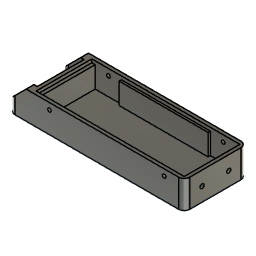
Upper Case v1 (Autodesk Fusion 360 design; units mm, degrees)
Autodesk Fusion 360 part; units mm, degrees
sketch "Sketch1" plane through (0, 0, 0) normal (0, 0, 1) x (1, 0, 0)
  line L0 (0, 0) -> (133, 0)
  line L1 (133, 0) -> (133, -56)
  line L2 (133, -56) -> (0, -56)
  line L3 (0, -56) -> (0, 0)
  dimension "d1" = 133
  dimension "d2" = 56
  constraint horizontal L0
  constraint vertical L1
  constraint horizontal L2
  constraint vertical L3
  constraint coincident L0.start L3.end
  measures "d1" distance of L0.start L0.end
  measures "d2" distance of L0.start L2.end
extrude "Extrude1" add sketch "Sketch1" along normal blind 3
sketch "Sketch2" plane through (0, 0, 3) normal (0, 0, 1) x (-1, 0, 0)
  line L0 (0, 56) -> (-133, 56)
  line L1 (-133, 56) -> (-133, 0)
  line L2 (-133, 0) -> (0, 0)
  line L3 (0, 0) -> (0, 56)
  line L4 (-3, 3) -> (-136, 3)
  line L5 (-136, 3) -> (-136, 53)
  line L6 (-136, 53) -> (-3, 53)
  line L7 (-3, 53) -> (-3, 3)
  dimension "d5" = 133
  dimension "d6" = 50
  dimension "d7" = 3
  dimension "d8" = 3
  constraint horizontal L4
  constraint vertical L5
  constraint horizontal L6
  constraint vertical L7
  measures "d5" distance of L4.start L4.end
  measures "d6" distance of L4.start L6.end
  measures "d7" distance of L2 L4
  measures "d8" distance of L3 L7
move_face "OffsetFaces1" offset 6 1 faces at (133, -18.6667, 1)
extrude "Extrude2" add sketch "Sketch2" along normal blind 22 contours L0 L1 L2 L3 L4 L6 L7
sketch "Sketch3" plane through (0, 0, 3) normal (0, 0, 1) x (-1, 0, 0)
  line L0 (-133, 0) -> (-133, 3)
  line L1 (-133, 3) -> (-3, 3)
  line L2 (-3, 3) -> (-3, 53)
  line L3 (-3, 53) -> (-133, 53)
  line L4 (-133, 53) -> (-133, 56)
  line L5 (-133, 56) -> (-139, 56)
  line L6 (-139, 56) -> (-139, 0)
  line L7 (-139, 0) -> (-133, 0)
  line L8 (-139, 0) -> (-136, 0)
  line L9 (-136, 0) -> (-136, 56)
  line L10 (-136, 56) -> (-139, 56)
  line L11 (-139, 56) -> (-139, 0)
  constraint horizontal L8
  constraint vertical L9
  constraint horizontal L10
  constraint vertical L11
  constraint midpoint L5 L9.end
  constraint coincident L6.end L7.start
extrude "Extrude3" add sketch "Sketch3" along normal blind 22 contours L5 L6 L7 L8 L9 L10 L11
move_face "OffsetFaces2" offset 5 1 faces at (133, -55, 10.3333)
move_face "OffsetFaces3" offset 5 1 faces at (133, -1, 17.6667)
sketch "Sketch4" plane through (0, 0, 0) normal (0, 1, 0) x (-1, 0, 0)
  line L0 (0, 25) -> (-139, 25)
  line L1 (-139, 25) -> (-139, 0)
  line L2 (-139, 0) -> (0, 0)
  line L3 (0, 0) -> (0, 25)
  line L4 (-136, 31.9366) -> (-136, -10) construction
  line L5 (-3, 30) -> (-3, -10) construction
  line L6 (-121, 35.1496) -> (-121, -13.3371) construction
  line L7 (-18, 34.1272) -> (-18, -18.3027) construction
  line L8 (-146.6322, 22) -> (13.2863, 22) construction
  line L9 (-145.902, 19.25) -> (3.6473, 19.25) construction
  point P0 (-121, 19.25)
  point P1 (-18, 19.25)
  dimension "d16" = 3
  dimension "d17" = 3
  dimension "d18" = 15
  dimension "d19" = 15
  dimension "d20" = 3
  dimension "d21" = 2.75
  constraint perpendicular L2 L4
  constraint perpendicular L2 L5
  constraint perpendicular L2 L6
  constraint perpendicular L0 L7
  constraint perpendicular L6 L8
  constraint perpendicular L3 L9
  constraint coincident L6 P0
  constraint coincident L9 P0
  constraint coincident L7 P1
  constraint coincident L9 P1
  measures "d16" distance of L1 L4
  measures "d17" distance of L3 L5
  measures "d18" distance of L4 L6
  measures "d19" distance of L5 L7
  measures "d20" distance of L0 L8
  measures "d21" distance of L8 L9
hole "Hole1" at (121, 0, 19.25) at (18, 0, 19.25) direction (0, -1, 0) diameter 3.3 depth 100 tip angle 118
sketch "Sketch5" plane through (0, 0, 3) normal (0, 0, 1) x (-1, 0, 0)
  line L0 (-136, 53) -> (-136, 3)
  line L1 (-136, 3) -> (-3, 3)
  line L2 (-3, 3) -> (-3, 53)
  line L3 (-3, 53) -> (-136, 53)
  line L4 (-3, 3) -> (-6, 3)
  line L5 (-6, 3) -> (-6, 53)
  line L6 (-6, 53) -> (-3, 53)
  line L7 (-3, 53) -> (-3, 3)
  line L8 (-136, 3) -> (-133, 3)
  line L9 (-133, 3) -> (-133, 53)
  line L10 (-133, 53) -> (-136, 53)
  line L11 (-136, 53) -> (-136, 3)
  line L12 (-69.5, -8.6587) -> (-69.5, 85) construction
  line L13 (0, 0) -> (0, 56) construction
  line L14 (-29.5, 3) -> (-109.5, 3)
  line L15 (-109.5, 3) -> (-109.5, 5)
  line L16 (-109.5, 5) -> (-29.5, 5)
  line L17 (-29.5, 5) -> (-29.5, 3)
  line L18 (-29.5, 53) -> (-109.5, 53)
  line L19 (-109.5, 53) -> (-109.5, 51)
  line L20 (-109.5, 51) -> (-29.5, 51)
  line L21 (-29.5, 51) -> (-29.5, 53)
  dimension "d25" = 3
  dimension "d26" = 3
  dimension "d27" = 69.5
  dimension "d28" = 80
  dimension "d29" = 2
  dimension "d30" = 80
  dimension "d31" = 2
  dimension "d32" = 40
  dimension "d33" = 40
  constraint horizontal L4
  constraint vertical L5
  constraint horizontal L6
  constraint vertical L7
  constraint coincident L1.end L2.start
  constraint horizontal L8
  constraint vertical L9
  constraint horizontal L10
  constraint vertical L11
  constraint coincident L0.end L1.start
  constraint perpendicular L1 L12
  constraint horizontal L14
  constraint vertical L15
  constraint horizontal L16
  constraint vertical L17
  constraint coincident L1 L14.start
  constraint horizontal L18
  constraint vertical L19
  constraint horizontal L20
  constraint vertical L21
  constraint coincident L3 L18.start
  measures "d25" distance of L1.end L4.end
  measures "d26" distance of L0.end L8.end
  measures "d27" distance of L12 L13
  measures "d28" distance of L14.start L14.end
  measures "d29" distance of L14.start L16.end
  measures "d30" distance of L18.start L18.end
  measures "d31" distance of L18.start L20.end
  measures "d32" distance of L12 L15
  measures "d33" distance of L12 L21
extrude "Extrude4" add sketch "Sketch5" along normal blind 19 contours L0 L1 L3 L8 L9 L10 L11 | L3 L18 L19 L20 L21 | L1 L14 L15 L16 L17 | L1 L2 L3 L4 L5 L6 L7
sketch "Sketch6" plane through (139, 0, 0) normal (1, 0, 0) x (0, 1, 0)
  line L0 (-56, 0) -> (0, 0)
  line L1 (0, 0) -> (0, 25)
  line L2 (0, 25) -> (-56, 25)
  line L3 (-56, 25) -> (-56, 0)
  line L4 (-28, 31.6217) -> (-28, -10) construction
  line L5 (-63.3305, 12.5) -> (7.7545, 12.5) construction
  line L6 (-40, 29.5194) -> (-40, -10) construction
  line L7 (-16, 30.045) -> (-16, -15) construction
  point P0 (-40, 12.5)
  point P1 (-16, 12.5)
  dimension "d36" = 28
  dimension "d37" = 12.5
  dimension "d38" = 12
  dimension "d39" = 12
  constraint perpendicular L0 L4
  constraint perpendicular L4 L5
  constraint perpendicular L2 L6
  constraint perpendicular L2 L7
  constraint coincident L5 P0
  constraint coincident L6 P0
  constraint coincident L5 P1
  constraint coincident L7 P1
  measures "d36" distance of L3 L4
  measures "d37" distance of L2 L5
  measures "d38" distance of L4 L6
  measures "d39" distance of L4 L7
hole "Hole2" at (139, -40, 12.5) at (139, -16, 12.5) direction (-1, 0, 0) diameter 3.75 depth 20 tip angle 118
sketch "Sketch7" plane through (0, 0, 0) normal (-1, 0, 0) x (0, -1, 0)
  line L0 (0, 0) -> (56, 0)
  line L1 (56, 0) -> (56, 25)
  line L2 (56, 25) -> (0, 25)
  line L3 (0, 25) -> (0, 0)
  line L4 (56, 0) -> (0, 0)
  line L5 (0, 0) -> (0, 7)
  line L6 (0, 7) -> (56, 7)
  line L7 (56, 7) -> (56, 0)
  dimension "d43" = 56
  dimension "d44" = 7
  constraint horizontal L4
  constraint vertical L5
  constraint horizontal L6
  constraint vertical L7
  constraint coincident L0.end L1.start
  measures "d43" distance of L0.end L0.start
  measures "d44" distance of L0.end L6.end
extrude "Extrude5" add sketch "Sketch7" along normal blind 18 contours L0 L1 L3 L4 L5 L6 L7
sketch "Sketch8" plane through (0, 0, 7) normal (0, 0, 1) x (-1, 0, 0)
  line L0 (0, 56) -> (0, 0)
  line L1 (0, 0) -> (18, 0)
  line L2 (18, 0) -> (18, 56)
  line L3 (18, 56) -> (0, 56)
  line L4 (18, 0) -> (0, 0)
  line L5 (0, 0) -> (0, 7)
  line L6 (0, 7) -> (18, 7)
  line L7 (18, 7) -> (18, 0)
  line L8 (18, 56) -> (0, 56)
  line L9 (0, 56) -> (0, 49)
  line L10 (0, 49) -> (18, 49)
  line L11 (18, 49) -> (18, 56)
  dimension "d47" = 7
  dimension "d48" = 7
  constraint horizontal L4
  constraint vertical L5
  constraint horizontal L6
  constraint vertical L7
  constraint coincident L1.end L2.start
  constraint horizontal L8
  constraint vertical L9
  constraint horizontal L10
  constraint vertical L11
  constraint coincident L2.end L3.start
  measures "d47" distance of L1.end L6.end
  measures "d48" distance of L2.end L10.end
extrude "Extrude6" add sketch "Sketch8" along normal blind 18 contours L0 L2 L3 L8 L9 L10 L11 | L0 L1 L2 L4 L5 L6 L7
chamfer "Chamfer1" distance 15 angle 45 2 edges at (-18, -3.5, 25) (-18, -52.5, 25)
sketch "Sketch9" plane through (0, 0, 7) normal (0, 0, 1) x (-1, 0, 0)
  line L0 (18, 49) -> (0, 49)
  line L1 (0, 49) -> (0, 7)
  line L2 (0, 7) -> (18, 7)
  line L3 (18, 7) -> (18, 49)
  line L4 (8.5413, 10) -> (6.5413, 10)
  line L5 (3.5413, 13) -> (3.5413, 43)
  line L6 (6.5413, 46) -> (8.5413, 46)
  line L7 (11.5413, 43) -> (11.5413, 13)
  line L8 (50, 28) -> (-30, 28) construction
  line L9 (3, 0) -> (18, 0) construction
  arc A0 (8.5413, 10) -> (11.5413, 13) centre (8.5413, 13) ccw
  arc A1 (3.5413, 13) -> (6.5413, 10) centre (6.5413, 13) ccw
  arc A2 (6.5413, 46) -> (3.5413, 43) centre (6.5413, 43) ccw
  arc A3 (11.5413, 43) -> (8.5413, 46) centre (8.5413, 43) ccw
  point P0 (11.5413, 10)
  point P1 (3.5413, 10)
  point P2 (11.5413, 46)
  dimension "d52" = 8
  dimension "d53" = 36
  dimension "d54" = 28
  dimension "d55" = 18
  dimension "d56" = 3
  constraint horizontal L4
  constraint vertical L5
  constraint horizontal L6
  constraint vertical L7
  constraint horizontal L8
  constraint coincident P0 L4
  constraint coincident P0 L7
  constraint tangent L4 A0
  constraint tangent L7 A0
  constraint coincident P1 L4
  constraint coincident P1 L5
  constraint tangent L4 A1
  constraint tangent L5 A1
  constraint equal A0 A1
  constraint tangent L5 A2
  constraint tangent L6 A2
  constraint equal A0 A2
  constraint coincident P2 L7
  constraint coincident P2 L6
  constraint tangent L7 A3
  constraint tangent L6 A3
  constraint equal A0 A3
  measures "d52" distance of P0 P1
  measures "d53" distance of P0 P2
  measures "d54" distance of L8 L9
  measures "d55" distance of L4 L8
  measures "d56" radius of A0
extrude "Extrude7" cut sketch "Sketch9" against normal blind 35 contours L4 L5 L6 L7 A0 A1 A2 A3
sketch "Sketch10" plane through (0, 0, 0) normal (0, 0, -1) x (1, 0, 0)
  line L0 (-11.5413, 13) -> (-11.5413, 43)
  arc A0 (-8.5413, 46) -> (-11.5413, 43) centre (-8.5413, 43) ccw
  line L1 (-8.5413, 46) -> (-6.5413, 46)
  arc A1 (-3.5413, 43) -> (-6.5413, 46) centre (-6.5413, 43) ccw
  line L2 (-3.5413, 43) -> (-3.5413, 13)
  arc A2 (-6.5413, 10) -> (-3.5413, 13) centre (-6.5413, 13) ccw
  line L3 (-6.5413, 10) -> (-8.5413, 10)
  arc A3 (-11.5413, 13) -> (-8.5413, 10) centre (-8.5413, 13) ccw
  line L4 (139, 56) -> (-18, 56)
  line L5 (-18, 56) -> (-18, 0)
  line L6 (-18, 0) -> (139, 0)
  line L7 (139, 0) -> (139, 56)
fillet "Fillet1" radius 5 1 edges at (139, -56, 12.5)
fillet "Fillet2" radius 5 2 edges at (139, 0, 12.5) (-18, 0, 5)
fillet "Fillet3" radius 5 1 edges at (-18, -56, 5)
fillet "Fillet4" radius 5 1 edges at (-18, -7, 8.5)
fillet "Fillet5" radius 5 1 edges at (-18, -49, 8.5)
